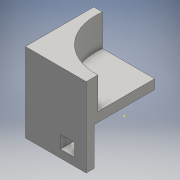
# Autodesk Inventor part: 240510_3Dsketch08
Saved by Autodesk Inventor 2016 (Build 200138000, 138)
## iProperties
Created: 2024-05-10
Part Number: 240510_3Dsketch08
Material: 일반
Document SubType Name: Modeling
Designer: pc
Density: 1 g/cm^3
Appearance: 기본값
Author: pc
Autodesk Inventor part; units mm, degrees
ref_plane "YZ Plane" through (0, 0, 0) normal (1, 0, 0) x (0, 1, 0)
ref_plane "XZ Plane" through (0, 0, 0) normal (0, 1, 0) x (-1, 0, 0)
ref_plane "XY Plane" through (0, 0, 0) normal (0, 0, 1) x (1, 0, 0)
sketch "스케치1" plane through (0, 0, 0) normal (0, 0, 1) x (1, 0, 0)
  line L0 (9.6169, -10.809) -> (-9.6169, -10.809)
  line L1 (-9.6169, -10.809) -> (-9.6169, 10.809)
  line L2 (-9.6169, 10.809) -> (9.6169, 10.809)
  line L3 (9.6169, 10.809) -> (9.6169, -10.809)
  line L4 (9.6169, -10.809) -> (-9.6169, 10.809) construction
  line L5 (-9.6169, -10.809) -> (9.6169, 10.809) construction
  point P0 (0, 0)
  constraints: 12 end point, 2 midpoint, 2 parallel, 1 horizontal, 1 perpendicular
extrude "돌출1" add sketch "스케치1" along normal blind 25
sketch "스케치2" plane through (-9.6169, 10.809, 0) normal (0, 1, 0) x (1, 0, 0)
  point P0 (9.6169, 0)
sketch "스케치3" plane through (0, 0, 25) normal (0, 0, 1) x (1, 0, 0)
  line L0 (9.6169, -10.809) -> (9.6169, 10.809) projected
  arc A0 (-6.8694, 10.809) -> (9.6169, -7.1319) centre (8.8168, 8.6782) ccw
  line L1 (-6.8694, 10.809) -> (9.6169, 10.809)
  point P0 (0, 0)
  constraints: 2 end point, 2 point on circle, 1 centre point, 1 horizontal, 1 point on line
extrude "돌출2" cut sketch "스케치3" against normal blind 10
sketch "스케치4" plane through (0, 0, 0) normal (0, 0, -1) x (-1, 0, 0)
  line L0 (9.6169, 10.809) -> (9.6169, -10.809) projected
  line L1 (9.6169, 10.809) -> (-9.6169, -8.323)
  line L2 (-9.6169, 10.809) -> (-9.6169, -10.809) projected
  line L3 (-9.6169, -8.323) -> (-9.6169, 10.809)
  line L4 (9.6169, 10.809) -> (-9.6169, 10.809) projected
  line L5 (9.6169, 10.809) -> (-9.6169, 10.809)
  point P0 (0, 0)
  constraints: 6 end point, 1 collinear, 1 horizontal, 1 point on line
sketch "스케치5" plane through (-9.6169, 10.809, 0) normal (0, 1, 0) x (1, 0, 0)
  line L0 (11.1073, -6.5575) -> (15.5096, -6.5575)
  line L1 (15.5096, -6.5575) -> (15.5096, -2.4763)
  line L2 (15.5096, -2.4763) -> (11.1073, -2.4763)
  line L3 (11.1073, -2.4763) -> (11.1073, -6.5575)
  line L4 (0, 0) -> (19.2339, 0) projected
  line L5 (0.0558, -2.4763) -> (5.1459, -2.4763)
  line L6 (5.1459, -2.4763) -> (5.1459, 0)
  line L7 (5.1459, 0) -> (0.0558, 0)
  line L8 (0.0558, 0) -> (0.0558, -2.4763)
  point P0 (9.6169, 0)
  constraints: 16 end point, 4 parallel, 2 horizontal, 2 perpendicular, 1 point on line
extrude "돌출3" cut sketch "스케치5" against normal blind 50 contours L3 L2 L1 L0
extrude "돌출4" cut sketch "스케치4" against normal blind 12
sketch "스케치6" plane through (-9.6169, -10.809, 25) normal (-1, 0, 0) x (0, 0, 1)
  line L0 (-25, 21.6179) -> (-13, 21.6179) projected
  line L1 (-25, 21.6179) -> (-21.9007, 21.6179)
  line L2 (-21.9007, 21.6179) -> (-21.9007, 17.0226)
  line L3 (-21.9007, 17.0226) -> (-25, 17.0226)
  line L4 (-25, 17.0226) -> (-25, 21.6179)
  point P0 (-25, 10.809)
  constraints: 8 end point, 2 parallel, 1 horizontal, 1 perpendicular
extrude "돌출5" cut sketch "스케치6" against normal blind 12
